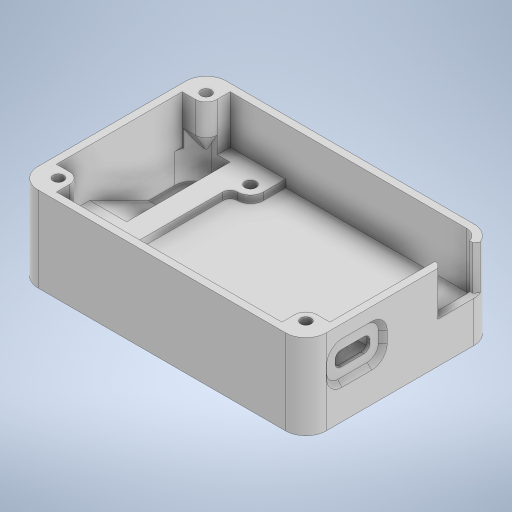
# Autodesk Inventor part: Main body
Saved by Autodesk Inventor 2023 (Build 270158000, 158)
## iProperties
Created: 2024-10-10
Part Number: Main body
Material: Generic
Document SubType Name: Modeling
Designer: noname
Density: 1 g/cm^3
Appearance: Default
Author: noname
Autodesk Inventor part; units mm, degrees
ref_plane "YZ Plane" through (0, 0, 0) normal (1, 0, 0) x (0, 1, 0)
ref_plane "XZ Plane" through (0, 0, 0) normal (0, 1, 0) x (-1, 0, 0)
ref_plane "XY Plane" through (0, 0, 0) normal (0, 0, 1) x (1, 0, 0)
sketch "Sketch1" plane through (0, 0, 0) normal (0, 1, 0) x (-1, 0, 0)
  line L0 (2.5, 0) -> (55, 0) construction
  line L1 (60, -5) -> (60, -40) construction
  line L2 (55, -45) -> (2.5, -45) construction
  line L3 (0, -42.5) -> (0, -2.5) construction
  arc A0 (2.5, 0) -> (0, -2.5) centre (2.5, -2.5) ccw construction
  arc A1 (0, -42.5) -> (2.5, -45) centre (2.5, -42.5) ccw construction
  arc A2 (55, -45) -> (60, -40) centre (55, -40) ccw construction
  arc A3 (60, -5) -> (55, 0) centre (55, -5) ccw construction
  line L4 (61, -40) -> (61, -5)
  arc A4 (61, -5) -> (55, 1) centre (55, -5) ccw
  line L5 (55, 1) -> (2.5, 1)
  arc A5 (2.5, 1) -> (-1, -2.5) centre (2.5, -2.5) ccw
  line L6 (-1, -2.5) -> (-1, -42.5)
  arc A6 (-1, -42.5) -> (2.5, -46) centre (2.5, -42.5) ccw
  line L7 (2.5, -46) -> (55, -46)
  arc A7 (55, -46) -> (61, -40) centre (55, -40) ccw
  line L8 (2.5, 3) -> (69.5, 3)
  line L9 (75, -2.5) -> (75, -42.5)
  line L10 (69.5, -48) -> (2.5, -48)
  arc A8 (-3, -42.5) -> (2.5, -48) centre (2.5, -42.5) ccw
  line L11 (-3, -42.5) -> (-3, -2.5)
  arc A9 (2.5, 3) -> (-3, -2.5) centre (2.5, -2.5) ccw
  arc A10 (69.5, -48) -> (75, -42.5) centre (69.5, -42.5) ccw
  arc A11 (75, -2.5) -> (69.5, 3) centre (69.5, -2.5) ccw
  point P0 (0, 0)
  point P1 (0, -45)
  dimension "d1" = 45
  dimension "d2" = 2.5
  dimension "d3" = 5
  dimension "d4" = 1
  dimension "d5" = 2
  dimension "d26" = 60
  dimension "d27" = 15
  constraints: 24 end point, 24 point on circle, 13 tangent, 12 centre point, 6 parallel, 4 equal radius, 4 point on line, 3 perpendicular, 1 horizontal, 10 other
  measures "d1" distance of point (0, -45) point (0, 0)
  measures "d2" radius of A0
  measures "d3" radius of A2
  measures "d4" distance between parallel lines of L0 L5
  measures "d5" distance between parallel lines of L8 L5
  measures "d26" distance between parallel lines of L3 L1
  measures "d27" distance between parallel lines of L1 L9
extrude "Extrusion1" add sketch "Sketch1" along normal blind 15
sketch "Sketch2" plane through (0, 0, 0) normal (0, -1, 0) x (1, 0, 0)
  line L0 (-2.5, -48) -> (-69.5, -48) projected
  arc A0 (-2.5, -48) -> (3, -42.5) centre (-2.5, -42.5) ccw projected
  line L1 (3, -2.5) -> (3, -42.5) projected
  arc A1 (3, -2.5) -> (-2.5, 3) centre (-2.5, -2.5) ccw projected
  line L2 (-69.5, 3) -> (-2.5, 3) projected
  arc A2 (-69.5, 3) -> (-75, -2.5) centre (-69.5, -2.5) ccw projected
  line L3 (-75, -42.5) -> (-75, -2.5) projected
  arc A3 (-75, -42.5) -> (-69.5, -48) centre (-69.5, -42.5) ccw projected
  arc A4 (-61, -40) -> (-55, -46) centre (-55, -40) ccw projected
  line L4 (-61, -5) -> (-61, -40) projected
  arc A5 (-55, 1) -> (-61, -5) centre (-55, -5) ccw projected
  line L5 (-2.5, 1) -> (-55, 1) projected
  arc A6 (1, -2.5) -> (-2.5, 1) centre (-2.5, -2.5) ccw projected
  line L6 (1, -42.5) -> (1, -2.5) projected
  arc A7 (-2.5, -46) -> (1, -42.5) centre (-2.5, -42.5) ccw projected
  line L7 (-55, -46) -> (-2.5, -46) projected
  point P0 (0, 0)
extrude "Extrusion2" add sketch "Sketch2" along normal blind 8 contours L0 A3 L3 A2 L2 A1 L1 A0 | L4 A5 L5 A6 L6 A7 L7 A4
sketch "Sketch3" plane through (0, 0, 0) normal (0, 1, 0) x (1, 0, 0)
  circle A0 centre (-26, 5) radius 1.5
  line L0 (-2.5, 0) -> (-55, 0) construction
  line L1 (0, 42.5) -> (0, 2.5) construction
  circle A1 centre (-55, 40) radius 1.5
  line L2 (-60, 5) -> (-60, 40) construction
  line L3 (-55, 45) -> (-2.5, 45) construction
  arc A2 (-22.5, 5) -> (-29.5, 5) centre (-26, 5) ccw
  line L4 (-22.5, 5) -> (-22.5, -1)
  line L5 (-2.5, -1) -> (-55, -1) construction
  line L6 (-29.5, 5) -> (-29.5, -1)
  arc A3 (-55, 36.5) -> (-51.5, 40) centre (-55, 40) ccw
  line L7 (-55, 36.5) -> (-55, 36.5)
  line L8 (-61, 5) -> (-61, 40) construction
  line L9 (-51.5, 40) -> (-51.5, 46)
  line L10 (-55, 46) -> (-2.5, 46) construction
  line L11 (-57, 34.5) -> (-57, -0.6569)
  arc A4 (-61, 5) -> (-55, -1) centre (-55, 5) ccw projected
  arc A5 (-61, 5) -> (-55, -1) centre (-55, 5) ccw projected
  line L12 (-8, -1) -> (-8, 16)
  line L13 (-6, 18) -> (1, 18)
  line L14 (1, 42.5) -> (1, 2.5) construction
  arc A6 (-6, 18) -> (-8, 16) centre (-6, 16) ccw
  arc A7 (-55, 36.5) -> (-57, 34.5) centre (-55, 34.5) ccw
  line L15 (-29.5, -1) -> (-22.5, -1)
  line L16 (-8, -1) -> (-2.5, -1)
  line L17 (1, 2.5) -> (1, 18)
  line L18 (-51.5, 46) -> (-55, 46)
  arc A8 (-2.5, -1) -> (1, 2.5) centre (-2.5, 2.5) ccw
  arc A9 (-61, 5) -> (-57, -0.6569) centre (-55, 5) ccw
  line L19 (-61, 5) -> (-61, 40)
  arc A10 (-55, 46) -> (-61, 40) centre (-55, 40) ccw
  point P0 (0, 0)
  point P1 (-61, 36.5)
  dimension "d11" = 5
  dimension "d12" = 26
  dimension "d13" = 5
  dimension "d14" = 5
  dimension "d15" = 3
  dimension "d16" = 3
  dimension "d17" = 3.5
  dimension "d18" = 3.5
  dimension "d20" = 3
  dimension "d21" = 2
  dimension "d22" = 18
  dimension "d23" = 8
  constraints: 24 end point, 16 point on circle, 11 tangent, 9 centre point, 7 point on line, 5 collinear, 3 vertical, 2 coincident, 2 horizontal, 2 perpendicular, 1 equal radius
  measures "d11" distance from line of L0 A0.centre
  measures "d12" distance from line of L1 A0.centre
  measures "d13" distance from line of L3 A1.centre
  measures "d14" distance from line of L2 A1.centre
  measures "d15" diameter of A1
  measures "d16" diameter of A0
  measures "d17" radius of A3
  measures "d18" radius of A2
  measures "d20" distance between parallel lines of L11 L2
  measures "d21" radius of A6
  measures "d22" distance between parallel lines of L0 L13
  measures "d23" distance between parallel lines of L1 L12
extrude "Extrusion3" add sketch "Sketch3" along normal blind 2
sketch "Sketch7" plane through (0, -8, 0) normal (0, -1, 0) x (1, 0, 0)
  circle A0 centre (-36, -22.5) radius 20
  line L0 (3, -42.5) -> (3, -2.5) projected
  line L1 (-69.5, -48) -> (-2.5, -48) projected
  point P0 (0, 0)
  point P1 (3, -22.5)
  point P2 (-36, -48)
  dimension "d29" = 40
  constraints: 2 midpoint, 1 centre point, 1 horizontal alignment, 1 vertical alignment
  measures "d29" diameter of A0
extrude "Extrusion4" cut sketch "Sketch7" against normal blind 2
sketch "Sketch8" plane through (-36, -6, -22.5) normal (0, -1, 0) x (1, 0, 0)
  circle A0 centre (0, 0) radius 15
  point P0 (36, 22.5)
  dimension "d32" = 30
  constraints: 1 centre point
  measures "d32" diameter of A0
extrude "Extrusion5" cut sketch "Sketch8" against normal blind 4.6
sketch "Sketch9" plane through (0, 15, 0) normal (0, 1, 0) x (1, 0, 0)
  line L0 (-2.5, 48) -> (-69.5, 48) projected
  arc A0 (-69.5, 48) -> (-75, 42.5) centre (-69.5, 42.5) ccw projected
  line L1 (-75, 42.5) -> (-75, 2.5) projected
  arc A1 (-75, 2.5) -> (-69.5, -3) centre (-69.5, 2.5) ccw projected
  line L2 (-69.5, -3) -> (-2.5, -3) projected
  arc A2 (-2.5, -3) -> (3, 2.5) centre (-2.5, 2.5) ccw projected
  line L3 (3, 2.5) -> (3, 42.5) projected
  arc A3 (3, 42.5) -> (-2.5, 48) centre (-2.5, 42.5) ccw projected
  arc A4 (-55, 46) -> (-61, 40) centre (-55, 40) ccw projected
  line L4 (-55, 46) -> (-2.5, 46) projected
  arc A5 (1, 42.5) -> (-2.5, 46) centre (-2.5, 42.5) ccw projected
  line L5 (1, 42.5) -> (1, 2.5) projected
  arc A6 (-2.5, -1) -> (1, 2.5) centre (-2.5, 2.5) ccw projected
  line L6 (-2.5, -1) -> (-55, -1) projected
  arc A7 (-61, 5) -> (-55, -1) centre (-55, 5) ccw projected
  line L7 (-61, 5) -> (-61, 40) projected
  line L8 (-55, -1) -> (-69.5, -1)
  line L9 (-73, 2.5) -> (-73, 42.5)
  line L10 (-55, 46) -> (-51.5, 46) projected
  line L11 (-69.5, 46) -> (-55, 46)
  line L12 (-69.5, 2.5) -> (-73.3891, -1.3891) construction
  arc A8 (-73, 2.5) -> (-69.5, -1) centre (-69.5, 2.5) ccw
  arc A9 (-69.5, 46) -> (-73, 42.5) centre (-69.5, 42.5) ccw
  point P0 (0, 0)
  point P1 (-73, -1)
  constraints: 8 end point, 5 point on circle, 4 tangent, 3 point on line, 2 centre point, 2 equal radius, 2 horizontal, 1 perpendicular
extrude "Extrusion6" cut sketch "Sketch9" against normal up to surface (13 mm away) contours A4 L7 A7 L8 A8 L9 A9 L11
sketch "Sketch10" plane through (-73, 15, -2.5) normal (1, 0, 0) x (0, 0, -1)
  line L0 (0, -13) -> (40, -13) projected
  line L1 (40, 0) -> (40, -13) projected
  line L2 (0, 0) -> (40, 0) projected
  line L3 (0, 0) -> (0, -13) projected
  line L4 (0, -23) -> (0, 0) projected
  line L5 (40, 0) -> (0, 0) projected
  line L6 (40, -23) -> (40, 0) projected
  line L7 (0, -23) -> (40, -23) projected
  line L8 (35, -16.4) -> (5, -16.4) projected
  line L9 (35, -21) -> (5, -21) projected
  line L10 (12, -13) -> (28, -21)
  line L11 (40, -21) -> (28, -21)
  line L12 (40, -21) -> (40, -13)
  line L13 (40, -13) -> (12, -13)
  point P0 (-2.5, -15)
  dimension "d38" = 12
  dimension "d39" = 12
  constraints: 8 end point, 4 point on line, 2 collinear, 1 perpendicular
  measures "d38" distance from line of L6 L10.end
  measures "d39" distance from line of L4 L10.start
extrude "Extrusion7" cut sketch "Sketch10" along normal blind 10 contours L0 L6 L11 L9 L10
sketch "Sketch11" plane through (-73, -6, -30.5) normal (0, 1, 0) x (1, 0, 0)
  line L0 (0, 0) -> (0, 12) projected
  line L1 (0, 0) -> (10, 0) projected
  line L2 (10, 0) -> (10, 12) projected
  line L3 (0, 12) -> (10, 12) projected
  circle A0 centre (37, -8) radius 15 projected
  circle A1 centre (37, -8) radius 20 projected
  circle A2 centre (37, -8) radius 15 projected
  line L4 (10, 12) -> (37, 12)
  line L5 (10, 12) -> (10, -16) projected
  line L6 (10, 0) -> (24.3114, 0)
  circle A3 centre (37, -8) radius 15 projected
  line L7 (29, 4.6886) -> (29, 12)
  point P0 (73, -30.5)
  point P1 (18.6697, 0)
  point P2 (29, 4.6886)
  dimension "d45" = 8
  constraints: 6 end point, 2 horizontal, 2 point on circle, 1 perpendicular, 1 point on line, 2 other
  measures "d45" distance from line of A0.centre L7
extrude "Extrusion8" cut sketch "Sketch11" along normal up to surface (4.6 mm away) contours L2 L4 L7 A1 L6 | A1 L7 A0 L6 | A0 picked at (24.3817, 5.1432)
chamfer "Chamfer1" distance 6 angle 45 2 edges at (-44, -3.7, -35.1886) (-48.6886, -3.7, -30.5)
sketch "Sketch12" plane through (-38.3871, -6, -37.3088) normal (-0.568605, 0, 0.8226107) x (0.8226107, 0, 0.568605)
  line L0 (-31.4247, 0) -> (-31.4247, 8) projected
  line L1 (-31.4247, 0) -> (-7.5689, 0) projected
  line L2 (-7.5689, 0) -> (-7.5689, 4.6) projected
  line L3 (-7.5689, 4.6) -> (-23.1985, 4.6) projected
  line L4 (-23.1985, 4.6) -> (-23.1985, 8) projected
  line L5 (-31.4247, 8) -> (-23.1985, 8) projected
  line L6 (-6.8233, 4.6) -> (-6.8233, 0) projected
  line L7 (-6.8233, 4.6) -> (-7.5689, 4.6) projected
  line L8 (-7.5689, 0) -> (-7.5689, 4.6) projected
  line L9 (-6.8233, 0) -> (-7.5689, 0) projected
  line L10 (-9.6968, 4.6) -> (-9.6968, 0)
  point P0 (52.7916, 6)
  point P1 (-7.5689, 0)
  constraints: 2 end point, 2 point on line, 1 perpendicular
extrude "Extrusion9" add sketch "Sketch12" against normal through all contours L10 L3 L2 L1 | L2 L7 L6 L9
fillet "Fillet1" radius 5 1 edges at (-73, -2, -42.5)
sketch "Sketch13" plane through (0, -6, 0) normal (0, -1, 0) x (1, 0, 0)
  circle A0 centre (-36, -22.5) radius 20 projected
  line L0 (-36, -22.5) -> (-21.8579, -8.3579) construction
  line L1 (-36, -22.5) -> (-30.8236, -41.8185) construction
  line L2 (-36, -22.5) -> (-55.3185, -17.3236) construction
  arc A1 (-55.9952, -22.9399) -> (-53.0964, -12.1215) centre (-56.1235, -17.1079) ccw
  arc A2 (-38.3871, -37.3088) -> (-50.8088, -24.8871) centre (-36, -22.5) ccw projected
  line L3 (3, -42.5) -> (3, -2.5) projected
  line L4 (-50.8088, -24.8871) -> (-54.4669, -30.1793) projected
  arc A3 (-38.3871, -37.3088) -> (-50.8088, -24.8871) centre (-36, -22.5) ccw projected
  line L5 (-43.6793, -40.9669) -> (-38.3871, -37.3088) projected
  arc A4 (-43.6793, -40.9669) -> (-54.4669, -30.1793) centre (-36, -22.5) ccw projected
  arc A5 (-25.6215, -39.5964) -> (-36.4399, -42.4952) centre (-30.6079, -42.6235) ccw
  arc A6 (-26.3833, -4.9638) -> (-18.4638, -12.8833) centre (-21.2686, -7.7686) ccw
  point P0 (0, 0)
  point P1 (-25.3934, -11.8934)
  point P2 (-26.3833, -4.9638)
  point P3 (-50.4889, -18.6177)
  point P4 (-18.4638, -12.8833)
  point P5 (-32.1177, -36.9889)
  point P6 (-25.6215, -39.5964)
  point P7 (-50.8088, -24.8871)
  dimension "d52" = 120
  dimension "d53" = 120
  dimension "d55" = 45
  dimension "d58" = 360
  constraints: 11 point on circle, 6 end point, 3 centre point, 1 point on line, 1 tangent, 14 other
  measures "d52" angle of L0 L2
  measures "d53" angle of L1 L2
  measures "d55" angle of L3 L0
extrude "Extrusion10" cut sketch "Sketch13" against normal up to surface (4.6 mm away) contours A0 A5 A2 A6 | A6 A2 A1 A0 | A0 L5 A2 A5 | A2 L4 A0 A1
sketch "Sketch14" plane through (0, -6, 0) normal (0, -1, 0) x (1, 0, 0)
  arc A0 (-55.9952, -22.9399) -> (-53.0964, -12.1215) centre (-56.1235, -17.1079) ccw projected
  arc A1 (-53.0964, -12.1215) -> (-55.9952, -22.9399) centre (-36, -22.5) ccw projected
  arc A2 (-25.6215, -39.5964) -> (-36.4399, -42.4952) centre (-30.6079, -42.6235) ccw projected
  arc A3 (-36.4399, -42.4952) -> (-25.6215, -39.5964) centre (-36, -22.5) ccw projected
  arc A4 (-26.3833, -4.9638) -> (-18.4638, -12.8833) centre (-21.2686, -7.7686) ccw projected
  arc A5 (-18.4638, -12.8833) -> (-26.3833, -4.9638) centre (-36, -22.5) ccw projected
  point P0 (0, 0)
extrude "Extrusion11" add sketch "Sketch14" along normal up to surface (2 mm away)
sketch "Sketch15" plane through (0, -8, 0) normal (0, -1, 0) x (1, 0, 0)
  line L0 (-45.8973, -42.5) -> (-43.6793, -40.9669) projected
  arc A0 (-43.6793, -40.9669) -> (-36.4399, -42.4952) centre (-36, -22.5) ccw projected
  arc A1 (-25.6215, -39.5964) -> (-36.4399, -42.4952) centre (-30.6079, -42.6235) ccw projected
  arc A2 (-25.6215, -39.5964) -> (-18.4638, -12.8833) centre (-36, -22.5) ccw projected
  arc A3 (-26.3833, -4.9638) -> (-18.4638, -12.8833) centre (-21.2686, -7.7686) ccw projected
  arc A4 (-26.3833, -4.9638) -> (-53.0964, -12.1215) centre (-36, -22.5) ccw projected
  arc A5 (-55.9952, -22.9399) -> (-53.0964, -12.1215) centre (-56.1235, -17.1079) ccw projected
  arc A6 (-55.9952, -22.9399) -> (-54.4669, -30.1793) centre (-36, -22.5) ccw projected
  line L1 (-54.6886, -30.5) -> (-54.4669, -30.1793) projected
  line L2 (-63, -30.5) -> (-54.6886, -30.5) projected
  line L3 (-63, -42.5) -> (-63, -30.5) projected
  line L4 (-45.8973, -42.5) -> (-63, -42.5) projected
  circle A7 centre (-36, -22.5) radius 18
  point P0 (0, 0)
  point P1 (-36.041, -40.5)
  point P2 (-26.9645, -38.0679)
  point P3 (-20.3911, -13.5356)
  point P4 (-27.0356, -6.8911)
  point P5 (-51.5679, -13.4645)
  point P6 (-54, -22.541)
  dimension "d64" = 36
  constraints: 1 centre point, 1 coincident
  measures "d64" diameter of A7
extrude "Extrusion12" cut sketch "Sketch15" against normal blind 2 contours A1 A7 | A7 A5 | A3 A7
chamfer "Chamfer2" distance 2 angle 45 3 edges at (-53.3867, -8, -17.8413) (-23.2721, -8, -9.7721) (-31.3413, -8, -39.8867)
sketch "Sketch16" plane through (0, 2, 0) normal (0, 1, 0) x (1, 0, 0)
  circle A0 centre (-55, 40) radius 1.5 projected
  line L0 (-68, 42.5) -> (-63, 42.5) projected
  line L1 (-63, 42.5) -> (-63, 14.5) projected
  line L2 (-63, 14.5) -> (-73, 14.5) projected
  line L3 (-73, 2.5) -> (-73, 14.5) projected
  arc A1 (-73, 2.5) -> (-69.5, -1) centre (-69.5, 2.5) ccw projected
  line L4 (-55, -1) -> (-69.5, -1) projected
  arc A2 (-57, -0.6569) -> (-55, -1) centre (-55, 5) ccw projected
  line L5 (-57, -0.6569) -> (-57, 34.5) projected
  arc A3 (-55, 36.5) -> (-57, 34.5) centre (-55, 34.5) ccw projected
  arc A4 (-55, 36.5) -> (-51.5, 40) centre (-55, 40) ccw projected
  line L6 (-51.5, 40) -> (-51.5, 46) projected
  line L7 (-69.5, 46) -> (-51.5, 46) projected
  arc A5 (-69.5, 46) -> (-73, 42.5) centre (-69.5, 42.5) ccw projected
  line L8 (-73, 37.5) -> (-73, 42.5) projected
  arc A6 (-68, 42.5) -> (-73, 37.5) centre (-68, 37.5) ccw projected
  arc A7 (-66.5, 2.5) -> (-69.5, 5.5) centre (-69.5, 2.5) ccw
  line L9 (-66.5, 2.5) -> (-66.5, -1)
  line L10 (-69.5, 5.5) -> (-73, 5.5)
  line L11 (-73, 5.5) -> (-73, 2.5)
  arc A8 (-73, 2.5) -> (-69.5, -1) centre (-69.5, 2.5) ccw projected
  line L12 (-69.5, -1) -> (-66.5, -1)
  arc A9 (-69.5, 39.5) -> (-66.5, 42.5) centre (-69.5, 42.5) ccw
  line L13 (-66.5, 42.5) -> (-66.5, 46)
  line L14 (-69.5, 39.5) -> (-73, 39.5)
  line L15 (-73, 39.5) -> (-73, 42.5)
  line L16 (-66.5, 46) -> (-69.5, 46)
  point P0 (0, 0)
  dimension "d70" = 3
  constraints: 16 end point, 5 point on circle, 5 tangent, 4 point on line, 3 vertical, 2 centre point, 2 coincident, 2 collinear, 2 perpendicular, 1 equal radius, 1 horizontal
  measures "d70" radius of A7
extrude "Extrusion13" add sketch "Sketch16" along normal up to surface (13 mm away) contours A6 L14 L8 A5 L7 L13 L0 | L0 A9 L14 A6 | L10 A7 L9 L4 A1 L3
chamfer "Chamfer3" distance 4.6 angle 30 2 edges at (-67.3787, 2, -40.3787) (-71.0413, 2, -39.5) measured on face at (-67.3787, 2.5, -40.3787) measured on face at (-71.0413, 2.5, -39.5)
sketch "Sketch17" plane through (0, 15, 0) normal (0, 1, 0) x (1, 0, 0)
  line L0 (-2.5, -1) -> (-66.5, -1) projected
  line L1 (-5.5, -1) -> (-5.5, 2.5)
  line L2 (-2.5, 5.5) -> (1, 5.5)
  line L3 (1, 42.5) -> (1, 2.5) projected
  arc A0 (-2.5, -3) -> (3, 2.5) centre (-2.5, 2.5) ccw projected
  arc A1 (-2.5, -1) -> (1, 2.5) centre (-2.5, 2.5) ccw projected
  arc A2 (-2.5, 5.5) -> (-5.5, 2.5) centre (-2.5, 2.5) ccw
  point P0 (0, 0)
  dimension "d76" = 3
  constraints: 4 end point, 2 point on circle, 2 point on line, 2 tangent, 1 centre point, 1 coincident, 1 perpendicular, 1 vertical
  measures "d76" radius of A2
extrude "Extrusion14" add sketch "Sketch17" against normal blind 10
sketch "Sketch18" plane through (1, 15, -5.5) normal (0, 0, -1) x (-1, 0, 0)
  line L0 (0, 0) -> (3.5, 0) projected
  line L1 (0, -10) -> (0, 0) projected
  line L2 (3.5, -10) -> (0, -10) projected
  line L3 (3.5, 0) -> (3.5, -10) projected
  line L4 (3.5, 0) -> (6.5, 0) projected
  line L5 (3.5, 0) -> (3.5, -10) projected
  line L6 (6.5, -10) -> (3.5, -10) projected
  line L7 (6.5, 0) -> (6.5, -10) projected
  line L8 (0, -13) -> (0, -10) projected
  line L9 (0, -10) -> (6.5, -3.5)
  point P0 (1, -15)
  dimension "d79" = 45
  constraints: 2 end point, 1 point on line
  measures "d79" angle of L1 L9
extrude "Extrusion15" cut sketch "Sketch18" against normal up to surface (6.5 mm away) contours L9 L3 L2 | L9 L7 L6 L3
sketch "Sketch20" plane through (-2.5, 5, 1) normal (0, 1, 0) x (1, 0, 0)
  arc A0 (0, 0) -> (3.5, 3.5) centre (0, 3.5) ccw projected
  line L0 (0, 0) -> (3.5, 0) projected
  line L1 (3.5, 3.5) -> (3.5, 0) projected
  point P0 (2.5, 1)
extrude "Extrusion16" add sketch "Sketch20" along normal through all
sketch "Sketch21" plane through (3, 15, -2.5) normal (1, 0, 0) x (0, 0, -1)
  line L0 (0, -13) -> (-3.5, -13) projected
  line L1 (-3.1569, -13) -> (-3.5, -13) projected
  line L2 (-3.1569, -13) -> (32, -13) projected
  line L3 (32, -13) -> (34, -13) projected
  line L4 (34, -13) -> (37.5, -13) projected
  line L5 (37.5, -13) -> (43.5, -13) projected
  line L6 (43.5, -13) -> (40, -13) projected
  line L7 (40, -13) -> (12, -13) projected
  line L8 (3, -13) -> (12, -13) projected
  line L9 (3, -13) -> (0, -13) projected
  line L10 (36, -13) -> (39, -13) projected
  line L11 (3.6, -11.2) -> (13, -11.2)
  line L12 (13, -11.2) -> (13, -7.2)
  line L13 (13, -7.2) -> (3.6, -7.2)
  line L14 (3.6, -7.2) -> (3.6, -11.2)
  line L15 (-3.5, -6.5) -> (-3.5, -13) projected
  line L16 (-3.5, -13) -> (-3.5, -15) projected
  line L17 (-3.5, -15) -> (-3.5, -13) projected
  line L18 (-3.5, -13) -> (-3.5, -15) projected
  line L19 (-3.5, -15) -> (-3.5, -13) projected
  line L20 (-3.5, -13) -> (-3.5, 0) projected
  line L21 (-3.5, 0) -> (-3.5, -3.5) projected
  line L22 (-3.5, -6.5) -> (-3.5, -3.5) projected
  line L23 (0, 0) -> (40, 0) projected
  line L24 (40, 0) -> (3, 0) projected
  point P0 (-2.5, -15)
  point P1 (21.5, 0)
  dimension "d84" = 1.8
  dimension "d85" = 5.8
  dimension "d86" = 9.4
  dimension "d90" = 8.5
  constraints: 8 end point, 2 parallel, 1 horizontal, 1 midpoint, 1 perpendicular
  measures "d84" distance between parallel lines of L2 L11
  measures "d85" distance between parallel lines of L2 L13
  measures "d86" distance between parallel lines of L12 L14
  measures "d90" distance from line of L12 point (21.5, 0)
extrude "Extrusion17" cut sketch "Sketch21" against normal up to surface (2 mm away)
fillet "Fillet2" radius 1.6 4 edges at (2, 3.8, -15.5) (2, 7.8, -15.5) (2, 7.8, -6.1) (2, 3.8, -6.1)
sketch "Sketch22" plane through (3, 15, -2.5) normal (1, 0, 0) x (0, 0, -1)
  line L0 (4.3, -4.7) -> (12.3, -4.7)
  line L1 (15.3, -7.7) -> (15.3, -10.7)
  line L2 (12.3, -13.7) -> (4.3, -13.7)
  line L3 (1.3, -10.7) -> (1.3, -7.7)
  arc A0 (4.3, -4.7) -> (1.3, -7.7) centre (4.3, -7.7) ccw
  arc A1 (15.3, -7.7) -> (12.3, -4.7) centre (12.3, -7.7) ccw
  arc A2 (12.3, -13.7) -> (15.3, -10.7) centre (12.3, -10.7) ccw
  arc A3 (1.3, -10.7) -> (4.3, -13.7) centre (4.3, -10.7) ccw
  line L4 (3.6, -9.6) -> (3.6, -8.8) projected
  line L5 (5.2, -7.2) -> (11.4, -7.2) projected
  point P0 (-2.5, -15)
  point P1 (8.3, -5.6)
  point P2 (8.3, -4.7)
  point P3 (2, -9.2)
  point P4 (1.3, -9.2)
  point P5 (3.6, -9.2)
  point P6 (8.3, -7.2)
  dimension "d95" = 9
  dimension "d96" = 14
  dimension "d97" = 3
  constraints: 8 end point, 8 point on circle, 8 tangent, 4 centre point, 4 midpoint, 3 equal radius, 2 horizontal alignment, 2 parallel, 2 vertical alignment, 1 horizontal, 1 perpendicular
  measures "d95" distance between parallel lines of L2 L0
  measures "d96" distance between parallel lines of L3 L1
  measures "d97" radius of A0
extrude "Extrusion18" cut sketch "Sketch22" against normal blind 1.2
chamfer "Chamfer5" distance 1.2 angle 45 8 edges at (3, 1.3, -10.8) (3, 2.1787, -4.6787) (3, 5.8, -3.8) (3, 9.4213, -4.6787) (3, 10.3, -10.8) (3, 9.4213, -16.9213) (3, 5.8, -17.8) (3, 2.1787, -16.9213)
sketch "Sketch23" plane through (3, 15, -2.5) normal (1, 0, 0) x (0, 0, -1)
  line L0 (31.4, 0) -> (41, 0)
  line L1 (41, 0) -> (41, -11.9)
  line L2 (41, -11.9) -> (31.4, -11.9)
  line L3 (31.4, -11.9) -> (31.4, 0)
  line L4 (0, -13) -> (-3.5, -13) projected
  line L5 (-3.1569, -13) -> (-3.5, -13) projected
  line L6 (-3.1569, -13) -> (32, -13) projected
  line L7 (32, -13) -> (34, -13) projected
  line L8 (34, -13) -> (37.5, -13) projected
  line L9 (37.5, -13) -> (43.5, -13) projected
  line L10 (43.5, -13) -> (40, -13) projected
  line L11 (40, -13) -> (12, -13) projected
  line L12 (3, -13) -> (12, -13) projected
  line L13 (3, -13) -> (0, -13) projected
  line L14 (36, -13) -> (39, -13) projected
  line L15 (0, 0) -> (40, 0) projected
  point P0 (-2.5, -15)
  point P1 (20, 0)
  dimension "d103" = 9.6
  dimension "d105" = 1.1
  dimension "d106" = 21
  constraints: 8 end point, 2 parallel, 1 horizontal, 1 midpoint, 1 perpendicular, 1 point on line
  measures "d103" distance between parallel lines of L1 L3
  measures "d105" distance between parallel lines of L11 L2
  measures "d106" distance from line of point (20, 0) L1
extrude "Extrusion19" cut sketch "Sketch23" against normal blind 10
chamfer "Chamfer6" distance 1.2 angle 45 2 edges at (3, 9.05, -33.9) (2.9083, 9.05, -43.5)
sketch "Sketch24" plane through (0, 15, 0) normal (0, 1, 0) x (1, 0, 0)
  arc A0 (-2.5, 5.5) -> (-5.5, 2.5) centre (-2.5, 2.5) ccw projected
  arc A1 (-66.5, 2.5) -> (-69.5, 5.5) centre (-69.5, 2.5) ccw projected
  arc A2 (-69.5, 39.5) -> (-66.5, 42.5) centre (-69.5, 42.5) ccw projected
  point P0 (0, 0)
  constraints: 3 coincident
hole "Hole1" at (-2.5, 15, -2.5) at (-69.5, 15, -2.5) at (-69.5, 15, -42.5) direction (0, -1, 0) diameter 2.8 depth 10 tip angle 118
body "Solid1"
